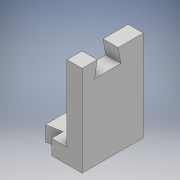
# Autodesk Inventor part: Frame VG01-2
Saved by Autodesk Inventor 2017 (Build 210142000, 142)
## iProperties
Created: 2019-03-04
Part Number: Frame VG01-2
Material: Generic
Document SubType Name: Modeling
Designer: Ben
Density: 1 g/cm^3
Appearance: Default
Author: Ben
Autodesk Inventor part; units mm, degrees
ref_plane "YZ Plane" through (0, 0, 0) normal (1, 0, 0) x (0, 1, 0)
ref_plane "XZ Plane" through (0, 0, 0) normal (0, 1, 0) x (-1, 0, 0)
ref_plane "XY Plane" through (0, 0, 0) normal (0, 0, 1) x (1, 0, 0)
sketch "Sketch1" plane through (0, 0, 0) normal (0, 1, 0) x (-1, 0, 0)
  line L0 (0, 0) -> (0, -35)
  line L1 (0, -35) -> (37, -35)
  line L2 (37, -35) -> (37, -55)
  line L3 (37, -55) -> (48, -55)
  line L4 (48, -55) -> (48, 0)
  line L5 (48, 0) -> (22, 0)
  line L6 (22, 0) -> (22, 0)
  line L7 (22, 0) -> (0, 0)
  dimension "d0" = 35
  dimension "d1" = 37
  dimension "d2" = 20
  dimension "d3" = 11
  dimension "d4" = 55
  dimension "d5" = 26
  dimension "d6" = 0
  constraints: 16 end point, 5 perpendicular, 2 vertical
  measures "d0" distance of L0.start L0.end
  measures "d1" distance of L0.end L1.end
  measures "d2" distance of L1.end L2.end
  measures "d3" distance of L2.end L3.end
  measures "d4" distance of L3.end L4.end
  measures "d5" distance of L4.end L5.end
  measures "d6" distance of L5.end L6.end
extrude "Extrusion1" add sketch "Sketch1" along normal blind 50
shell "Shell1" thickness 5 removed faces 3 at (-48, 16.6667, -36.6667) at (-19.6667, 0, -23.3333) at (-19.6667, 50, -23.3333)
sketch "Sketch2" plane through (0, 0, 0) normal (1, 0, 0) x (0, 0, -1)
  line L0 (5, 0) -> (30, 0) projected
  line L1 (5, 0) -> (19, 0)
  line L2 (19, 0) -> (19, 17)
  line L3 (19, 17) -> (5, 17)
  line L4 (5, 17) -> (5, 0)
  point P0 (0, 0)
  dimension "d10" = 17
  dimension "d11" = 0
  dimension "d12" = 11
  constraints: 8 end point, 2 parallel, 1 horizontal, 1 perpendicular, 1 point on line
  measures "d10" distance of L2.end L1.end
  measures "d11" distance from line of L4 L0.start
  measures "d12" distance from line of L2 L0.end
extrude "Extrusion2" cut sketch "Sketch2" against normal blind 10
sketch "Sketch3" plane through (-48, 0, -55) normal (-1, 0, 0) x (0, 0, 1)
  line L0 (0, 0) -> (0, 50) projected
  line L1 (5, 50) -> (25, 50) projected
  line L2 (0, 0) -> (5, 0)
  line L3 (5, 0) -> (5, 50)
  line L4 (5, 50) -> (0, 50)
  line L5 (0, 50) -> (0, 0)
  point P0 (55, 0)
  constraints: 8 end point, 2 parallel, 1 horizontal, 1 perpendicular
extrude "Extrusion3" add sketch "Sketch3" along normal blind 15
sketch "Sketch4" plane through (-48, 0, 0) normal (-1, 0, 0) x (0, 0, 1)
  line L0 (-5, 0) -> (0, 0) projected
  line L1 (-5, 0) -> (-5, 50) projected
  line L2 (0, 0) -> (-5, 0)
  line L3 (-5, 0) -> (-5, 50)
  line L4 (-5, 50) -> (0, 50)
  line L5 (0, 50) -> (0, 0)
  point P0 (0, 0)
  constraints: 8 end point, 2 parallel, 1 horizontal, 1 perpendicular
extrude "Extrusion4" add sketch "Sketch4" along normal blind 15
sketch "Sketch5" plane through (0, 17, -5) normal (0, 0, -1) x (-1, 0, 0)
  circle A0 centre (11.5, -8.5) radius 2.0828
  line L0 (63, -17) -> (0, -17) projected
  line L1 (0, -17) -> (0, 0) projected
  dimension "d19" = 4.1656
  dimension "d20" = 8.5
  dimension "d21" = 11.5
  constraints: 1 centre point
  measures "d19" diameter of A0
  measures "d20" distance from line of L0 A0.centre
  measures "d21" distance from line of L1 A0.centre
extrude "Extrusion5" cut sketch "Sketch5" against normal blind 15
sketch "Sketch6" plane through (0, 17, -5) normal (0, 0, -1) x (-1, 0, 0)
  circle A0 centre (28.505, 18.46) radius 2.0828
  line L0 (63, -17) -> (0, -17) projected
  line L1 (5, 0) -> (5, 33) projected
  dimension "d24" = 4.1656
  dimension "d25" = 35.46
  dimension "d26" = 23.505
  constraints: 1 centre point
  measures "d24" diameter of A0
  measures "d25" distance from line of L0 A0.centre
  measures "d26" distance from line of L1 A0.centre
extrude "Extrusion6" cut sketch "Sketch6" against normal blind 15
sketch "Sketch7" plane through (0, 17, -5) normal (0, 0, -1) x (-1, 0, 0)
  circle A0 centre (58.5, 19) radius 2.0828
  line L0 (63, 33) -> (63, -17) projected
  line L1 (5, 33) -> (63, 33) projected
  point P0 (0, -17)
  dimension "d29" = 4.1656
  dimension "d30" = 4.5
  dimension "d31" = 14
  constraints: 1 centre point
  measures "d29" diameter of A0
  measures "d30" distance from line of A0.centre L0
  measures "d31" distance from line of L1 A0.centre
extrude "Extrusion7" cut sketch "Sketch7" against normal blind 15
sketch "Sketch13" plane through (0, 0, -35) normal (0, 0, -1) x (-1, 0, 0)
  circle A0 centre (11.5, 8.5) radius 2.0828
  line L0 (0, 0) -> (37, 0) projected
  line L1 (0, 0) -> (0, 50) projected
  dimension "d41" = 4.1656
  dimension "d42" = 8.5
  dimension "d43" = 11.5
  constraints: 1 centre point
  measures "d41" diameter of A0
  measures "d42" distance from line of L0 A0.centre
  measures "d43" distance from line of L1 A0.centre
extrude "Extrusion9" cut sketch "Sketch13" against normal blind 15
sketch "Sketch14" plane through (-37, 0, -55) normal (0, 0, -1) x (-1, 0, 0)
  circle A0 centre (-8.495, 35.46) radius 2.0828
  line L0 (-37, 0) -> (-37, 50) projected
  line L1 (0, 0) -> (26, 0) projected
  dimension "d46" = 4.1656
  dimension "d47" = 28.505
  dimension "d48" = 35.46
  constraints: 1 centre point
  measures "d46" diameter of A0
  measures "d47" distance from line of L0 A0.centre
  measures "d48" distance from line of L1 A0.centre
extrude "Extrusion10" cut sketch "Sketch14" against normal blind 15
sketch "Sketch15" plane through (-37, 0, -55) normal (0, 0, -1) x (-1, 0, 0)
  circle A0 centre (21.5, 36) radius 2.0828
  line L0 (0, 0) -> (26, 0) projected
  line L1 (26, 50) -> (26, 0) projected
  point P0 (-37, 0)
  dimension "d51" = 4.1656
  dimension "d52" = 36
  dimension "d53" = 4.5
  constraints: 1 centre point
  measures "d51" diameter of A0
  measures "d52" distance from line of L0 A0.centre
  measures "d53" distance from line of L1 A0.centre
extrude "Extrusion11" cut sketch "Sketch15" against normal blind 15
sketch "Sketch16" plane through (-42, 0, -30) normal (-1, 0, 0) x (0, 0, 1)
  line L0 (0, 0) -> (-5, 0)
  line L1 (-5, 0) -> (-5, 50)
  line L2 (-5, 50) -> (0, 50)
  line L3 (0, 50) -> (0, 0)
  point P0 (30, 0)
  dimension "d56" = 5
  dimension "d57" = 50
  constraints: 8 end point, 2 parallel, 1 horizontal, 1 perpendicular
  measures "d56" distance of L1.end L2.end
  measures "d57" distance of L0.end L1.end
extrude "Extrusion12" add sketch "Sketch16" along normal blind 21
sketch "Sketch17" plane through (-5, 0, -30) normal (0, 0, 1) x (1, 0, 0)
  circle A0 centre (-23.505, 35.46) radius 2.0828
  line L0 (0, 0) -> (0, 50) projected
  line L1 (0, 0) -> (-58, 0) projected
  point P0 (5, 0)
  dimension "d60" = 4.1656
  dimension "d61" = 23.505
  dimension "d62" = 35.46
  constraints: 1 centre point
  measures "d60" diameter of A0
  measures "d61" distance from line of A0.centre L0
  measures "d62" distance from line of L1 A0.centre
extrude "Extrusion13" cut sketch "Sketch17" against normal blind 10
sketch "Sketch18" plane through (-42, 0, -35) normal (0, 0, -1) x (-1, 0, 0)
  circle A0 centre (16.5, 36) radius 2.0828
  line L0 (21, 50) -> (21, 0) projected
  line L1 (0, 0) -> (21, 0) projected
  point P0 (-42, 0)
  dimension "d65" = 4.1656
  dimension "d67" = 36
  dimension "d70" = 4.5
  constraints: 1 centre point
  measures "d65" diameter of A0
  measures "d67" distance from line of L1 A0.centre
  measures "d70" distance from line of L0 A0.centre
extrude "Extrusion14" cut sketch "Sketch18" against normal blind 10
sketch "Sketch20" plane through (-63, 0, 0) normal (-1, 0, 0) x (0, 0, 1)
  line L0 (0, 0) -> (-5, 0) projected
  line L1 (-5, 17) -> (-5, 50) projected
  line L2 (0, 0) -> (-5, 0)
  line L3 (-5, 0) -> (-5, 50)
  line L4 (-5, 50) -> (0, 50)
  line L5 (0, 50) -> (0, 0)
  constraints: 8 end point, 2 parallel, 1 horizontal, 1 perpendicular
extrude "Extrusion15" add sketch "Sketch20" along normal blind 2.583
sketch "Sketch21" plane through (-63, 0, -30) normal (-1, 0, 0) x (0, 0, 1)
  line L0 (-20, 50) -> (-5, 50) projected
  line L1 (11, 0) -> (0, 0) projected
  line L2 (-5, 50) -> (0, 50)
  line L3 (0, 50) -> (0, 0)
  line L4 (0, 0) -> (-5, 0)
  line L5 (-5, 0) -> (-5, 50)
  point P0 (30, 0)
  constraints: 8 end point, 2 parallel, 1 horizontal, 1 perpendicular
extrude "Extrusion16" add sketch "Sketch21" along normal blind 2.583
sketch "Sketch22" plane through (-63, 0, -55) normal (-1, 0, 0) x (0, 0, 1)
  line L0 (0, 0) -> (0, 50) projected
  line L1 (5, 0) -> (5, 50) projected
  line L2 (0, 50) -> (5, 50)
  line L3 (5, 50) -> (5, 0)
  line L4 (5, 0) -> (0, 0)
  line L5 (0, 0) -> (0, 50)
  point P0 (55, 0)
  constraints: 8 end point, 2 parallel, 1 horizontal, 1 perpendicular
extrude "Extrusion17" add sketch "Sketch22" along normal blind 2.583
sketch "Sketch23" plane through (0, 0, 0) normal (0, 0, 1) x (1, 0, 0)
  line L0 (0, 50) -> (-37, 50) projected
  line L1 (-65.583, 50) -> (-65.583, 0) projected
  line L2 (0, 50) -> (-65.583, 50)
  line L3 (-65.583, 50) -> (-65.583, 43.083)
  line L4 (-65.583, 43.083) -> (0, 43.083)
  line L5 (0, 43.083) -> (0, 50)
  point P0 (0, 0)
  dimension "d77" = 6.917
  constraints: 8 end point, 2 parallel, 1 horizontal, 1 perpendicular, 1 point on line
  measures "d77" distance of L4.end L0.start
extrude "Extrusion18" cut sketch "Sketch23" against normal blind 100
sketch "Sketch24" plane through (0, 0, -35) normal (0, 0, -1) x (-1, 0, 0)
  line L0 (0, 0) -> (65.583, 0) projected
  line L1 (31.0052, 0) -> (26.0052, 0)
  line L2 (26.0052, 5) -> (31.0052, 5)
  circle A0 centre (28.505, 35.46) radius 2.0828 projected
  line L3 (26.0052, 5) -> (25.0052, 5)
  line L4 (25.0052, 5) -> (26.0052, 0)
  line L5 (31.0052, 5) -> (32.0052, 5)
  line L6 (32.0052, 5) -> (31.0052, 0)
  dimension "d80" = 5
  dimension "d81" = 5
  dimension "d83" = 1
  dimension "d84" = 1
  constraints: 12 end point, 3 horizontal, 1 parallel, 1 point on line
  measures "d80" distance of L2.start L2.end
  measures "d81" distance of L1.end L2.start
  measures "d83" distance of L2.start L3.end
  measures "d84" distance of L2.end L5.end
extrude "Extrusion19" cut sketch "Sketch24" against normal blind 100 contours L4 L3 L2 L5 L6 L0
sketch "Sketch25" plane through (0, 0, 0) normal (1, 0, 0) x (0, 0, -1)
  line L0 (0, 0) -> (5, 0) projected
  line L1 (35, 43.083) -> (0, 43.083) projected
  line L2 (0, 0) -> (5, 0)
  line L3 (5, 0) -> (5, 43.083)
  line L4 (5, 43.083) -> (0, 43.083)
  line L5 (0, 43.083) -> (0, 0)
  dimension "d87" = 5
  constraints: 8 end point, 2 parallel, 1 horizontal, 1 perpendicular, 1 point on line
  measures "d87" distance of L4.end L3.end
extrude "Extrusion20" cut sketch "Sketch25" against normal blind 100
sketch "Sketch26" plane through (0, 0, -19) normal (1, 0, 0) x (0, 0, -1)
  line L0 (-9, 35.6451) -> (-9, 26.9508)
  line L1 (-9, 26.9508) -> (-14, 27.8324)
  line L2 (-9, 35.6451) -> (-14, 34.7635)
  line L3 (-9, 35.6451) -> (-3.9229, 35.6451) construction
  line L4 (-14, 34.7635) -> (-14, 27.8324)
  line L5 (-14, 43.083) -> (-14, 17) projected
  line L6 (-14, 17) -> (0, 17) projected
  line L7 (16, 43.083) -> (-14, 43.083) projected
  point P0 (0, 0)
  dimension "d90" = 8.6943
  dimension "d91" = 80
  dimension "d92" = 170
  dimension "d93" = 0
  dimension "d94" = 5
  dimension "d128" = 7.4379
  constraints: 10 end point, 1 equal length, 1 horizontal, 1 parallel
  measures "d90" distance of L0.start L0.end
  measures "d91" angle of L0 L1
  measures "d92" angle of L2 L3
  measures "d93" distance between parallel lines of L5 L4
  measures "d94" distance between parallel lines of L0 L4
  measures "d128" distance from line of L7 L0.start
extrude "Extrusion21" cut sketch "Sketch26" against normal blind 100
sketch "Sketch27" plane through (-37, 0, -35) normal (1, 0, 0) x (0, 0, -1)
  line L0 (5, 17) -> (5, 8.3057)
  line L1 (5, 8.3057) -> (0, 9.1873)
  line L2 (5, 17) -> (0, 16.1184)
  line L3 (5, 17) -> (10.0771, 17) construction
  line L4 (0, 16.1184) -> (0, 9.1873)
  line L5 (0, 0) -> (0, 43.083) projected
  line L6 (20, 43.083) -> (0, 43.083) projected
  dimension "d98" = 8.6943
  dimension "d99" = 80
  dimension "d100" = 170
  dimension "d102" = 5
  dimension "d104" = 0
  dimension "d105" = 26.083
  constraints: 10 end point, 1 equal length, 1 horizontal, 1 parallel
  measures "d98" distance of L0.start L0.end
  measures "d99" angle of L0 L1
  measures "d100" angle of L2 L3
  measures "d102" distance between parallel lines of L0 L4
  measures "d104" distance between parallel lines of L5 L4
  measures "d105" distance from line of L6 L0.start
sketch "Sketch28" plane through (-37, 0, -35) normal (1, 0, 0) x (0, 0, -1)
  line L0 (5, 34.3887) -> (5, 25.6944)
  line L1 (5, 25.6944) -> (0, 26.576)
  line L2 (5, 34.3887) -> (0, 33.507)
  line L3 (5, 34.3887) -> (10.0771, 34.3887) construction
  line L4 (0, 33.507) -> (0, 26.576)
  dimension "d106" = 8.6943
  dimension "d107" = 80
  dimension "d108" = 170
  dimension "d109" = 5
  constraints: 10 end point, 1 equal length, 1 horizontal, 1 parallel
  measures "d106" distance of L0.start L0.end
  measures "d107" angle of L0 L1
  measures "d108" angle of L2 L3
  measures "d109" distance between parallel lines of L0 L4
extrude "Extrusion22" add sketch "Sketch27" along normal blind 5
extrude "Extrusion23" add sketch "Sketch28" along normal blind 5
sketch "Sketch29" plane through (-65.583, 43.083, -30) normal (0, 1, 0) x (1, 0, 0)
  line L0 (33.583, 5) -> (28.583, 5) projected
  line L1 (0, 25) -> (28.583, 25) projected
  line L2 (28.583, 5) -> (0, 5)
  line L3 (0, 5) -> (0, 25)
  line L4 (0, 25) -> (28.583, 25)
  line L5 (28.583, 25) -> (28.583, 5)
  point P0 (65.583, -30)
  constraints: 8 end point, 2 parallel, 1 horizontal, 1 perpendicular
extrude "Extrusion24" cut sketch "Sketch29" against normal blind 100
sketch "Sketch31" plane through (-65.583, 43.083, -30) normal (0, 0, 1) x (1, 0, 0)
  line L0 (60.583, -8.3195) -> (60.583, 0) projected
  line L1 (60.583, 0) -> (-3.7083, 0)
  line L2 (-3.7083, 0) -> (-3.7083, -46.9701)
  line L3 (-3.7083, -46.9701) -> (60.583, -46.9701)
  line L4 (60.583, -46.9701) -> (60.583, 0)
  point P0 (65.583, -43.083)
  constraints: 8 end point, 2 parallel, 1 horizontal, 1 perpendicular
extrude "Extrusion25" cut sketch "Sketch31" against normal blind 100
sketch "Sketch32" plane through (0, 0, -35) normal (0, 0, -1) x (-1, 0, 0)
  line L0 (10, 34.3887) -> (10, 25.6944)
  line L1 (10, 25.6944) -> (5, 26.576)
  line L2 (10, 34.3887) -> (5, 33.507)
  line L3 (10, 34.3887) -> (15.0771, 34.3887) construction
  line L4 (5, 33.507) -> (5, 26.576)
  line L5 (5, 0) -> (5, 43.083) projected
  line L6 (5, 43.083) -> (0, 43.083) projected
  dimension "d120" = 8.6943
  dimension "d121" = 80
  dimension "d122" = 170
  dimension "d123" = 5
  dimension "d124" = 0
  dimension "d125" = 8.6943
  constraints: 10 end point, 1 equal length, 1 horizontal, 1 parallel
  measures "d120" distance of L0.start L0.end
  measures "d121" angle of L0 L1
  measures "d122" angle of L2 L3
  measures "d123" distance between parallel lines of L0 L4
  measures "d124" distance between parallel lines of L5 L4
  measures "d125" distance from line of L6 L0.start
extrude "Extrusion26" add sketch "Sketch32" against normal blind 5
sketch "Sketch33" plane through (0, 0, -19) normal (1, 0, 0) x (0, 0, -1)
  line L0 (0, 0) -> (16, 0) projected
  line L1 (16, 0) -> (-15.3687, 0)
  line L2 (-15.3687, 0) -> (-15.3687, 22.832)
  line L3 (-15.3687, 22.832) -> (16, 22.832)
  line L4 (16, 22.832) -> (16, 0)
  point P0 (-19, 0)
  dimension "d130" = 22.832
  constraints: 8 end point, 2 parallel, 1 horizontal, 1 perpendicular
  measures "d130" distance of L1.end L2.end
extrude "Extrusion27" cut sketch "Sketch33" against normal blind 10
sketch "Sketch34" plane through (-10, 25.6944, -35) normal (-1, 0, 0) x (0, 0, 1)
  line L0 (0, -2.8624) -> (30, -2.8624) projected
  line L1 (0, 17.3886) -> (30, 17.3886) projected
  line L2 (0, -2.8624) -> (5, -2.8624)
  line L3 (5, -2.8624) -> (5, 17.3886)
  line L4 (5, 17.3886) -> (0, 17.3886)
  line L5 (0, 17.3886) -> (0, -2.8624)
  point P0 (35, -25.6944)
  dimension "d133" = 5
  constraints: 8 end point, 2 parallel, 1 horizontal, 1 perpendicular, 1 point on line
  measures "d133" distance of L4.end L3.end
extrude "Extrusion28" add sketch "Sketch34" against normal blind 5
sketch "Sketch35" plane through (0, 43.083, -35) normal (0, 0, -1) x (-1, 0, 0)
  line L0 (10, -20.251) -> (10, 0) projected
  line L1 (10, -16.507) -> (14.9999, -17.3886)
  line L2 (10, -16.507) -> (15.077, -16.507) construction
  line L3 (14.9999, -17.3886) -> (14.9999, -8.6944)
  line L4 (14.9999, -8.6944) -> (10, -9.576)
  line L5 (10, -9.576) -> (10, -16.507)
  point P0 (0, -43.083)
  dimension "d136" = 5.077
  dimension "d137" = 10
  dimension "d138" = 5.077
  dimension "d139" = 3.744
  dimension "d140" = 6.931
  constraints: 10 end point, 2 point on line, 1 collinear, 1 equal length, 1 horizontal, 1 parallel
  measures "d136" distance of L1.start L1.end
  measures "d137" angle of L1 L2
  measures "d138" distance of L3.end L4.end
  measures "d139" distance of L0.start L1.start
  measures "d140" distance of L4.end L1.start
extrude "Extrusion29" add sketch "Sketch35" against normal blind 5
body "Solid1"
